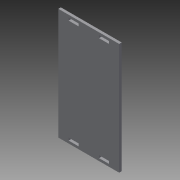
# Autodesk Inventor part: bottomPanel01
Saved by Autodesk Inventor 2013 (Build 170138000, 138)
## iProperties
Created: 2014-10-07
Part Number: bottomPanel01
Material: Generic
Document SubType Name: Modeling
Designer: Nano
Density: 1 g/cm^3
Author: Nano
Autodesk Inventor part; units mm, degrees
ref_plane "YZ Plane" through (0, 0, 0) normal (1, 0, 0) x (0, 1, 0)
ref_plane "XZ Plane" through (0, 0, 0) normal (0, 1, 0) x (-1, 0, 0)
ref_plane "XY Plane" through (0, 0, 0) normal (0, 0, 1) x (1, 0, 0)
sketch "Sketch1" plane through (0, 0, 0) normal (0, 0, 1) x (1, 0, 0)
  line L0 (-34.9814, 266.7) -> (-34.9814, -12.7) projected
  line L1 (-34.9814, -12.7) -> (117.4186, -12.7) projected
  line L2 (117.4186, -12.7) -> (117.4186, 266.7) projected
  line L3 (117.4186, 266.7) -> (-34.9814, 266.7) projected
  line L4 (177.4504, 254) -> (177.4504, 260.35) projected
  line L5 (177.4504, 260.35) -> (152.0504, 260.35) projected
  line L6 (152.0504, 260.35) -> (152.0504, 254) projected
  line L7 (152.0504, 254) -> (177.4504, 254) projected
  line L8 (101.2504, 254) -> (101.2504, 260.35) projected
  line L9 (101.2504, 260.35) -> (75.8504, 260.35) projected
  line L10 (75.8504, 260.35) -> (75.8504, 254) projected
  line L11 (75.8504, 254) -> (101.2504, 254) projected
  line L12 (177.4504, -6.35) -> (177.4504, 0) projected
  line L13 (177.4504, 0) -> (152.0504, 0) projected
  line L14 (152.0504, 0) -> (152.0504, -6.35) projected
  line L15 (152.0504, -6.35) -> (177.4504, -6.35) projected
  line L16 (101.2504, -6.35) -> (101.2504, 0) projected
  line L17 (101.2504, 0) -> (75.8504, 0) projected
  line L18 (75.8504, 0) -> (75.8504, -6.35) projected
  line L19 (75.8504, -6.35) -> (101.2504, -6.35) projected
  point P0 (0, 0)
extrude "Extrusion1" add sketch "Sketch1" along normal blind 6.35 contours L3 L2 L1 L0
body "Solid1"
